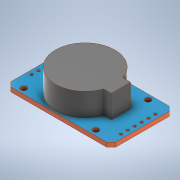
# Autodesk Inventor part: DS3231_RTC
Saved by Autodesk Inventor 2020.2 (Build 242310000, 310)
## iProperties
Created: 2020-04-10
Part Number: DS3231_RTC
Material: Phenolic Resin
Document SubType Name: Modeling
Designer: agmlego
Mass: 6.85369 g
Surface Area: 27.5779 cm^2
Volume: 4.96644 cm^3
Density: 1.38 g/cm^3
Appearance: Smooth - Light Orange
Author: agmlego
Autodesk Inventor part; units mm, degrees
ref_plane "YZ Plane" through (0, 0, 0) normal (1, 0, 0) x (0, 1, 0)
ref_plane "XZ Plane" through (0, 0, 0) normal (0, 1, 0) x (-1, 0, 0)
ref_plane "XY Plane" through (0, 0, 0) normal (0, 0, 1) x (1, 0, 0)
sketch "Sketch1" plane through (0, 0, 0) normal (0, 1, 0) x (-1, 0, 0)
  line L0 (1.6, 0) -> (37, 0)
  line L1 (38.6, -1.6) -> (38.6, -21.4)
  line L2 (37, -23) -> (1.6, -23)
  line L3 (0, -21.4) -> (0, -1.6)
  line L4 (0, -1.6) -> (1.6, 0)
  line L5 (37, 0) -> (38.6, -1.6)
  line L6 (38.6, -21.4) -> (37, -23)
  line L7 (0, -21.4) -> (1.6, -23)
  point P0 (0, 0)
  point P1 (38.6, -23)
  point P2 (38.6, 0)
  point P3 (0, -23)
  dimension "d0" = 23
  dimension "d1" = 38.6
  dimension "d2" = 1.6
  dimension "d3" = 1.6
  dimension "d4" = 1.6
  dimension "d5" = 1.6
  dimension "d6" = 1.6
  dimension "d7" = 1.6
  dimension "d8" = 1.6
  dimension "d9" = 1.6
  constraints: 16 end point, 8 point on line, 2 parallel, 1 horizontal, 1 perpendicular
  measures "d0" distance of point (0, -23) point (0, 0)
  measures "d1" distance of point (0, 0) point (38.6, 0)
  measures "d2" distance of L3.end point (0, 0)
  measures "d3" distance of L0.start point (0, 0)
  measures "d4" distance of L0.end point (38.6, 0)
  measures "d5" distance of L1.start point (38.6, 0)
  measures "d6" distance of L1.end point (38.6, -23)
  measures "d7" distance of L2.start point (38.6, -23)
  measures "d8" distance of L3.start point (0, -23)
  measures "d9" distance of L2.end point (0, -23)
extrude "PCB" add sketch "Sketch1" along normal blind 1.6
sketch "Sketch2" plane through (0, 1.6, 0) normal (0, 1, 0) x (1, 0, 0)
  line L0 (0, 1.6) -> (0, 21.4) projected
  line L1 (-37, 0) -> (-1.6, 0) projected
  circle A0 centre (-7.53, 1.89) radius 1.05 construction
  line L2 (-1.6, 23) -> (-37, 23) construction
  point P0 (0, 0)
  point P1 (-7.53, 21.11)
  point P2 (-34.05, 1.89)
  dimension "d12" = 7.53
  dimension "d13" = 1.89
  dimension "d14" = 2.1
  dimension "d15" = 1.89
  dimension "d16" = 34.05
  constraints: 1 centre point, 1 coincident, 1 horizontal alignment, 1 vertical alignment
  measures "d12" distance from line of L0 point (-7.53, 1.89)
  measures "d13" distance from line of L1 point (-7.53, 1.89)
  measures "d14" diameter of A0
  measures "d15" distance from line of L2 point (-7.53, 21.11)
  measures "d16" distance from line of L0 point (-34.05, 1.89)
hole "Mounting" at (-7.53, 1.6, -1.89) at (-7.53, 1.6, -21.11) at (-34.05, 1.6, -1.89) direction (0, -1, 0) diameter 2.1 end through all start extended yes
sketch "Sketch3" plane through (0, 1.6, 0) normal (0, 1, 0) x (1, 0, 0)
  line L0 (-38.6, 21.4) -> (-38.6, 1.6) construction
  line L1 (0, 1.6) -> (0, 21.4) construction
  line L2 (-37, 10.23) -> (-38.6, 11.5) construction
  line L3 (-37, 12.77) -> (-38.6, 11.5) construction
  line L4 (-1.6, 10.23) -> (0, 11.5) construction
  line L5 (0, 1.6) -> (0, 21.4) construction
  line L6 (-1.6, 12.77) -> (0, 11.5) construction
  point P0 (0, 0)
  point P1 (-1.6, 5.15)
  point P2 (-37, 7.69)
  point P3 (-37, 15.31)
  point P4 (-1.6, 7.69)
  point P5 (-1.6, 15.31)
  point P6 (-1.6, 17.85)
  dimension "d26" = 2.54
  dimension "d33" = 2.54
  dimension "d38" = 1.6
  dimension "d39" = 1.6
  constraints: 8 end point, 2 equal length, 2 midpoint, 2 vertical, 8 other
  measures "d26" distance of point (-37, 7.69) L2.start
  measures "d33" distance of point (-1.6, 5.15) point (-1.6, 7.69)
  measures "d38" distance from line of L1 point (-1.6, 5.15)
  measures "d39" distance from line of L0 point (-37, 7.69)
hole "0.1\" Pin Headers" at (-1.6, 1.6, -5.15) at (-37, 1.6, -7.69) at (-37, 1.6, -10.23) at (-37, 1.6, -12.77) at (-37, 1.6, -15.31) at (-1.6, 1.6, -7.69) at (-1.6, 1.6, -10.23) at (-1.6, 1.6, -12.77) at (-1.6, 1.6, -15.31) at (-1.6, 1.6, -17.85) direction (0, -1, 0) diameter 1.016 end through all start extended yes
sketch "Sketch14" plane through (0, 1.6, 0) normal (0, 1, 0) x (1, 0, 0)
  arc A0 (-10.73, 15.05) -> (-10.73, 7.95) centre (-21.078, 11.5) ccw
  line L0 (-10.73, 7.95) -> (-7.9, 7.95)
  line L1 (-7.9, 7.95) -> (-7.9, 15.05)
  line L2 (-7.9, 15.05) -> (-10.73, 15.05)
  line L3 (0, 1.6) -> (0, 21.4) projected
  line L4 (-7.9, 11.5) -> (0, 11.5) construction
  line L5 (0, 1.6) -> (0, 21.4) construction
  point P0 (0, 0)
  dimension "d47" = 21.88
  dimension "d48" = 7.1
  dimension "d49" = 2.83
  dimension "d50" = 7.9
  constraints: 8 end point, 3 perpendicular, 2 midpoint, 2 point on circle, 1 centre point, 1 horizontal, 1 parallel
  measures "d47" diameter of A0
  measures "d48" distance of L0.end L1.end
  measures "d49" distance of L1.end L2.end
  measures "d50" distance between parallel lines of L3 L1
extrude "CR2032 Holder" add sketch "Sketch14" along normal blind 8.5
sketch "Sketch15" plane through (0, 0, 0) normal (0, -1, 0) x (1, 0, 0)
  line L0 (-27.65, -19.1) -> (-17.35, -19.1)
  line L1 (-17.35, -19.1) -> (-17.35, -11.6)
  line L2 (-17.35, -11.6) -> (-27.65, -11.6)
  line L3 (-27.65, -11.6) -> (-27.65, -19.1)
  line L4 (-22.1, -6.4) -> (-17.1, -6.4)
  line L5 (-17.1, -6.4) -> (-17.1, -2.6)
  line L6 (-17.1, -2.6) -> (-22.1, -2.6)
  line L7 (-22.1, -2.6) -> (-22.1, -6.4)
  line L8 (-1.6, -23) -> (-37, -23) construction
  line L9 (-37, 0) -> (-1.6, 0) construction
  line L10 (-38.6, -21.4) -> (-38.6, -1.6) construction
  point P0 (0, 0)
  dimension "d53" = 10.3
  dimension "d54" = 7.5
  dimension "d55" = 5
  dimension "d56" = 3.8
  dimension "d57" = 3.9
  dimension "d58" = 2.6
  dimension "d59" = 10.95
  dimension "d60" = 16.5
  constraints: 16 end point, 4 parallel, 2 horizontal, 2 perpendicular
  measures "d53" distance of L0.start L0.end
  measures "d54" distance of L0.end L1.end
  measures "d55" distance of L5.end L6.end
  measures "d56" distance of L4.end L5.end
  measures "d57" distance between parallel lines of L8 L0
  measures "d58" distance between parallel lines of L9 L6
  measures "d59" distance between parallel lines of L10 L3
  measures "d60" distance between parallel lines of L10 L7
extrude "DS3231SN" add sketch "Sketch15" along normal blind 2.75 contours L3 L2 L1 L0
extrude "24C32N" add sketch "Sketch15" along normal blind 1.5 contours L7 L6 L5 L4
sketch "Sketch4" plane through (0, 0, 0) normal (0, -1, 0) x (1, 0, 0)
  circle A0 centre (-37, -7.69) radius 0.508 construction
sketch "Sketch5" plane through (0, 0, 0) normal (0, -1, 0) x (1, 0, 0)
  circle A0 centre (-37, -10.23) radius 0.508 construction
sketch "Sketch6" plane through (0, 0, 0) normal (0, -1, 0) x (1, 0, 0)
  circle A0 centre (-37, -12.77) radius 0.508 construction
sketch "Sketch7" plane through (0, 0, 0) normal (0, -1, 0) x (1, 0, 0)
  circle A0 centre (-37, -15.31) radius 0.508 construction
sketch "Sketch8" plane through (0, 0, 0) normal (0, -1, 0) x (1, 0, 0)
  circle A0 centre (-1.6, -5.15) radius 0.508 construction
sketch "Sketch9" plane through (0, 0, 0) normal (0, -1, 0) x (1, 0, 0)
  circle A0 centre (-1.6, -7.69) radius 0.508 construction
sketch "Sketch10" plane through (0, 0, 0) normal (0, -1, 0) x (1, 0, 0)
  circle A0 centre (-1.6, -10.23) radius 0.508 construction
sketch "Sketch11" plane through (0, 0, 0) normal (0, -1, 0) x (1, 0, 0)
  circle A0 centre (-1.6, -12.77) radius 0.508 construction
sketch "Sketch12" plane through (0, 0, 0) normal (0, -1, 0) x (1, 0, 0)
  circle A0 centre (-1.6, -15.31) radius 0.508 construction
sketch "Sketch13" plane through (0, 0, 0) normal (0, -1, 0) x (1, 0, 0)
  circle A0 centre (-1.6, -17.85) radius 0.508 construction
equation "\"d3\" = d2"
equation "\"d4\" = d2"
equation "\"d5\" = d4"
equation "\"d6\" = d2"
equation "\"d7\" = d6"
equation "\"d8\" = d2"
equation "\"d9\" = d8"
equation "\"d15\" = d13"
equation "\"d17\" = d14"
body "Solid1"
